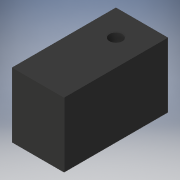
# Autodesk Inventor part: Motor
Saved by Autodesk Inventor 2019 (Build 230136000, 136)
## iProperties
Created: 2019-03-05
Part Number: Motor
Material: 일반
Document SubType Name: Modeling
Designer: Jeong Ji Hoon
Density: 1 g/cm^3
Appearance: 기본값
Author: Jeong Ji Hoon
Autodesk Inventor part; units mm, degrees
ref_plane "YZ Plane" through (0, 0, 0) normal (1, 0, 0) x (0, 1, 0)
ref_plane "XZ Plane" through (0, 0, 0) normal (0, 1, 0) x (-1, 0, 0)
ref_plane "XY Plane" through (0, 0, 0) normal (0, 0, 1) x (1, 0, 0)
sketch "스케치1" plane through (0, 0, 0) normal (0, 1, 0) x (-1, 0, 0)
  line L0 (0, 0) -> (40, 0)
  line L1 (40, 0) -> (40, -80)
  line L2 (40, -80) -> (0, -80)
  line L3 (0, -80) -> (0, 0)
  dimension "d0" = 40
  dimension "d1" = 80
  constraints: 8 end point, 2 parallel, 1 horizontal, 1 perpendicular
  measures "d0" distance of L1.end L2.end
  measures "d1" distance of L0.end L1.end
extrude "돌출1" add sketch "스케치1" along normal blind 50
sketch "스케치2" plane through (0, 50, 0) normal (0, 1, 0) x (1, 0, 0)
  line L0 (0, 80) -> (-40, 80) construction
  line L1 (-20, 80) -> (-20, 0) construction
  line L2 (-40, 0) -> (0, 0) construction
  point P0 (-20, 60)
  dimension "d4" = 20
  constraints: 2 end point, 2 midpoint, 1 point on line
  measures "d4" distance from line of point (-20, 60) L0
hole "구멍1" at (-20, 50, -60) direction (0, -1, 0) diameter 10 end through all
